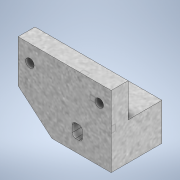
# Autodesk Inventor part: Soporte Idler Z
Saved by Autodesk Inventor 2021 (Build 250183000, 183)
## iProperties
Created: 2023-01-20
Part Number: Soporte Idler Z
Material: Hormigón reforzado con fibra de vidrio
Document SubType Name: Modeling
Designer: Diego.labarca
Density: 1.7 g/cm^3
Appearance: Plano - Pulido Gris
Author: Diego.labarca
Autodesk Inventor part; units mm, degrees
ref_plane "YZ Plane" through (0, 0, 0) normal (1, 0, 0) x (0, 1, 0)
ref_plane "XZ Plane" through (0, 0, 0) normal (0, 1, 0) x (-1, 0, 0)
ref_plane "XY Plane" through (0, 0, 0) normal (0, 0, 1) x (1, 0, 0)
sketch "Boceto1" plane through (0, 0, 0) normal (0, 0, 1) x (1, 0, 0)
  line L0 (-27.5, 10) -> (27.5, 10)
  line L1 (27.5, 10) -> (27.5, -10)
  line L2 (27.5, -10) -> (-27.5, -10)
  line L3 (-27.5, -10) -> (-27.5, 10)
  line L4 (0, 0) -> (0, 1.7227)
  line L5 (0, 0) -> (-2.1619, 0)
  line L6 (27.5, -10) -> (-2.5, -10)
  line L7 (-2.5, -10) -> (-2.5, -27)
  line L8 (-2.5, -27) -> (27.5, -27)
  line L9 (27.5, -27) -> (27.5, -10)
  circle A0 centre (20.5, 0) radius 2.5
  circle A1 centre (-20.5, 0) radius 2.5
  point P0 (-2.5, -10)
  dimension "d14" = 55
  dimension "d15" = 20
  dimension "d16" = 30
  dimension "d17" = 17
  dimension "d18" = 5
  dimension "d19" = 5
  dimension "d20" = 7
  dimension "d21" = 7
  constraints: 20 end point, 4 parallel, 3 horizontal, 2 centre point, 2 perpendicular, 1 vertical, 2 other
  measures "d14" distance of L1.end L2.end
  measures "d15" distance of L0.end L1.end
  measures "d16" distance of L8.end L7.end
  measures "d17" distance of L7.end L6.end
  measures "d18" diameter of A0
  measures "d19" diameter of A1
  measures "d20" distance from line of A0.centre L1
  measures "d21" distance from line of L3 A1.centre
extrude "Extrusión1" add sketch "Boceto1" along normal blind 10
sketch "Boceto2" plane through (-2.5, -27, 0) normal (0, -1, 0) x (1, 0, 0)
  line L0 (30, 10) -> (-25, 10) projected
  line L1 (30, 10) -> (0, 10)
  line L2 (0, 10) -> (0, -20)
  line L3 (0, -20) -> (30, -20)
  line L4 (30, -20) -> (30, 10)
  line L5 (0, 0) -> (0, 10) projected
  point P0 (2.5, 0)
  point P1 (0, 10)
  dimension "d22" = 30
  constraints: 8 end point, 2 parallel, 1 collinear, 1 horizontal, 1 perpendicular
  measures "d22" distance of L2.end L1.end
extrude "Extrusión2" add sketch "Boceto2" along normal blind 5
sketch "Boceto4" plane through (-27.5, -10, 0) normal (-1, 0, 0) x (0, 0, 1)
  line L0 (0, 0) -> (0, -17) projected
  line L1 (10, 20) -> (10, 0) projected
  line L2 (10, 0) -> (-20, 0)
  line L3 (-20, 0) -> (-20, -5)
  line L4 (-20, -5) -> (10, -5)
  line L5 (10, -5) -> (10, 0)
  line L6 (10, -22) -> (-20, -22) projected
  point P0 (0, 10)
  dimension "d32" = 5
  dimension "d43" = 30
  dimension "d44" = 30
  constraints: 8 end point, 2 parallel, 1 horizontal, 1 perpendicular
  measures "d32" distance of L3.end L2.end
  measures "d43" distance of L6.start L6.end
  measures "d44" distance of L3.end L4.end
extrude "Extrusión4" add sketch "Boceto4" against normal up to surface (55 mm away)
sketch "Boceto5" plane through (-2.5, -32, 0) normal (0, -1, 0) x (1, 0, 0)
  circle A0 centre (10, -9) radius 2.5
  line L0 (30, -20) -> (30, 10) projected
  line L1 (0, -20) -> (30, -20) projected
  line L2 (-25, -20) -> (30, -20) projected
  line L3 (-25, -20) -> (-25, 10) projected
  line L4 (-25, 0) -> (30, 0) projected
  point P0 (2.5, 0)
  point P1 (0, 0)
  dimension "d33" = 5
  dimension "d34" = 20
  dimension "d41" = 9
  constraints: 1 centre point
  measures "d33" diameter of A0
  measures "d34" distance from line of L0 A0.centre
  measures "d41" vertical distance of A0.centre point (0, 0)
extrude "Extrusión5" cut sketch "Boceto5" against normal up to surface (22 mm away) contours A0
sketch "Boceto8" plane through (-27.5, -15, -20) normal (0, -1, 0) x (1, 0, 0)
  line L0 (0, 30) -> (25, 30) projected
  line L1 (0, 0) -> (55, 0) projected
  line L2 (25, 30) -> (20, 30)
  line L3 (20, 30) -> (20, 0)
  line L4 (20, 0) -> (25, 0)
  line L5 (25, 0) -> (25, 30)
  line L6 (25, 20) -> (55, 20) projected
  line L7 (45, 20) -> (55, 20)
  line L8 (55, 20) -> (55, 0)
  line L9 (55, 0) -> (45, 0)
  line L10 (45, 0) -> (45, 20)
  line L11 (55, 0) -> (55, 20) projected
  point P0 (27.5, 20)
  point P1 (45, 0)
  point P2 (25, 0)
  point P3 (20, 30)
  dimension "d54" = 5
  dimension "d56" = 0
  dimension "d69" = 10
  constraints: 16 end point, 4 parallel, 3 point on line, 2 horizontal, 2 perpendicular
  measures "d54" distance of L4.end L3.end
  measures "d56" distance between parallel lines of L11 L8
  measures "d69" distance between parallel lines of L11 L10
extrude "Extrusión8" add sketch "Boceto8" along normal up to surface (17 mm away) contours L0 L5 L1 L3 | L6 L8 L1 L10
sketch "Boceto9" plane through (0, 0, 10) normal (0, 0, 1) x (1, 0, 0)
  line L0 (27.5, -32) -> (-7.5, -32) projected
  line L1 (-27.5, 10) -> (-27.5, -15) projected
  line L2 (-7.5, -32) -> (-27.5, -15)
  line L3 (-27.5, -15) -> (-7.5, -15) projected
  line L4 (-7.5, -15) -> (-7.5, -32) projected
  point P0 (0, 0)
  constraints: 2 end point
extrude "Extrusión9" add sketch "Boceto9" against normal up to surface (30 mm away)
sketch "Boceto10" plane through (-2.5, -32, 0) normal (0, -1, 0) x (1, 0, 0)
  circle A0 centre (-18, -9) radius 2.5
  line L0 (-25, 10) -> (-5, 10) projected
  line L1 (-25, -20) -> (-25, 10) projected
  point P0 (2.5, 0)
  dimension "d61" = 5
  dimension "d62" = 19
  dimension "d63" = 7
  constraints: 1 centre point
  measures "d61" diameter of A0
  measures "d62" distance from line of L0 A0.centre
  measures "d63" distance from line of L1 A0.centre
extrude "Extrusión10" cut sketch "Boceto10" against normal up to surface (22 mm away)
sketch "Boceto11" plane through (-2.5, -32, 0) normal (0, -1, 0) x (1, 0, 0)
  circle A0 centre (-18, -9) radius 2.5 projected
  circle A1 centre (-18, -9) radius 5
  point P0 (2.5, 0)
  dimension "d66" = 10
  constraints: 1 centre point, 1 coincident
  measures "d66" diameter of A1
extrude "Extrusión11" cut sketch "Boceto11" against normal blind 14 contours A0 | A1
sketch "Boceto12" plane through (0, 0, 10) normal (0, 0, 1) x (1, 0, 0)
  line L0 (7.5, -25) -> (4.5, -25)
  line L1 (4.5, -25) -> (4.5, -17)
  line L2 (4.5, -17) -> (7.5, -17)
  line L3 (7.5, -17) -> (7.5, -25)
  line L4 (7.5, -17) -> (10.5, -17)
  line L5 (10.5, -17) -> (10.5, -25)
  line L6 (7.5, -25) -> (7.5, -17)
  line L7 (27.5, -32) -> (-7.5, -32) projected
  line L8 (7.5, -25) -> (10.5, -25)
  line L9 (-27.5, -10) -> (27.5, -10) projected
  point P0 (0, 0)
  dimension "d70" = 3
  dimension "d72" = 3
  dimension "d77" = 7
  dimension "d78" = 8
  constraints: 16 end point, 4 parallel, 2 horizontal, 2 perpendicular, 1 collinear
  measures "d70" distance of L1.end L2.end
  measures "d72" distance from line of L4.end L3
  measures "d77" distance between parallel lines of L7 L0
  measures "d78" distance of L4.end L5.end
extrude "Extrusión12" cut sketch "Boceto12" against normal up to surface (10 mm away)
fillet "Empalme4" radius 2 4 edges at (10.5, -17, 5) (4.5, -17, 5) (10.5, -25, 5) (4.5, -25, 5)
equation "\"d19\" = d18"
equation "\"d20\" = d21"
equation "\"d44\" = d43"
equation "\"d72\" = d70"
